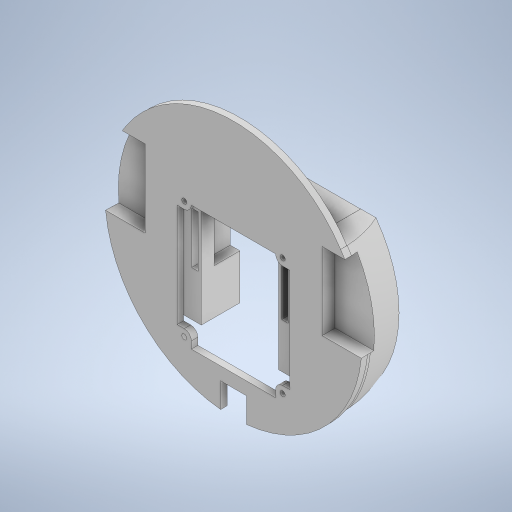
# Autodesk Inventor part: Wabbit
Saved by Autodesk Inventor 2024.2 (Build 282272000, 272)
## iProperties
Created: 2025-11-06
Part Number: Wabbit
Material: Generic
Document SubType Name: Modeling
Designer: David Toler II
Density: 1 g/cm^3
Appearance: Default
Author: David Toler II
Autodesk Inventor part; units mm, degrees
ref_plane "YZ Plane" through (0, 0, 0) normal (1, 0, 0) x (0, 1, 0)
ref_plane "XZ Plane" through (0, 0, 0) normal (0, 1, 0) x (-1, 0, 0)
ref_plane "XY Plane" through (0, 0, 0) normal (0, 0, 1) x (1, 0, 0)
sketch "Sketch1" plane through (0, 0, 0) normal (0, 0, 1) x (1, 0, 0)
  line L0 (27.78125, -44.45) -> (-27.78125, -44.45)
  line L1 (-27.78125, -44.45) -> (-27.78125, 44.45)
  line L2 (-27.78125, 44.45) -> (27.78125, 44.45)
  line L3 (27.78125, 44.45) -> (27.78125, -44.45)
  line L4 (27.78125, -44.45) -> (-27.78125, 44.45) construction
  line L5 (-27.78125, -44.45) -> (27.78125, 44.45) construction
  point P0 (0, 0)
  dimension "d0" = 88.9
  dimension "d1" = 55.5625
  constraints: 12 end point, 2 midpoint, 2 parallel, 1 horizontal, 1 perpendicular
  measures "d0" distance of L0.end L1.end
  measures "d1" distance of L0.start L0.end
extrude "Extrusion1" add sketch "Sketch1" along normal blind 25.4
sketch "Sketch2" plane through (0, 0, 0) normal (1, 0, 0) x (0, 1, 0)
  line L0 (44.45, 0) -> (-44.45, 0)
  line L1 (-44.45, 0) -> (-44.45, 25.4)
  line L2 (44.45, 25.4) -> (-44.45, 25.4)
  line L3 (44.45, 0) -> (44.45, 25.4)
  circle A0 centre (0, 0) radius 63.416389
  line L4 (-63.416389, 0) -> (0, 0)
  line L5 (0, 0) -> (0, 63.416389)
  line L6 (-63.416389, 0) -> (-51.195337, 0)
  line L7 (-54.624765, 25.4) -> (54.624765, 25.4)
  line L8 (54.624765, 25.4) -> (54.624765, 0)
  line L9 (54.624765, 0) -> (-54.624765, 0)
  line L10 (-54.624765, 0) -> (-54.624765, 25.4)
  circle A1 centre (0, 0) radius 60.241389
  line L11 (63.33686, -3.175) -> (-63.33686, -3.175)
  line L12 (0, -3.175) -> (0, 0)
  line L13 (54.624765, 0) -> (63.416389, 0)
  line L14 (-54.624765, 0) -> (-63.416389, 0)
  point P0 (-44.45, 0)
  point P1 (0, 25.4)
  point P2 (44.45, 0)
  dimension "d6" = 109.24953
  dimension "d7" = 3.175
  dimension "d12" = 3.175
  constraints: 22 end point, 6 point on circle, 4 midpoint, 3 perpendicular, 3 point on line, 2 collinear, 2 horizontal, 2 parallel, 1 centre point, 1 coincident, 1 vertical, 3 other
  measures "d6" distance between parallel lines of L8 L10
  measures "d12" distance between parallel lines of L11 L0
revolve "Revolution1" add sketch "Sketch2" angle 360 about axis through (0, 0, 0) along (0, 0, 1) contours L9 L13 A1 L11 L12 L0 | L13 A0 L11 A1
sketch "Sketch6" plane through (0, 0, 0) normal (0, 0, 1) x (1, 0, 0)
  circle A0 centre (0, 0) radius 63.416389
  line L0 (27.78125, -44.45) -> (27.78125, 44.45)
  line L1 (-27.78125, -44.45) -> (27.78125, -44.45)
  line L2 (-27.78125, 44.45) -> (-27.78125, -44.45)
  line L3 (27.78125, 44.45) -> (-27.78125, 44.45)
  line L4 (24.28125, -40.95) -> (24.28125, 40.95)
  line L5 (24.28125, 40.95) -> (-24.28125, 40.95)
  line L6 (-24.28125, 40.95) -> (-24.28125, -40.95)
  line L7 (-24.28125, -40.95) -> (24.28125, -40.95)
  circle A1 centre (-24.28125, -40.95) radius 1.25
  circle A2 centre (24.28125, -40.95) radius 1.25
  line L8 (-24.28125, 17.05) -> (24.28125, 17.05)
  circle A3 centre (-24.28125, 17.05) radius 1.25
  circle A4 centre (24.28125, 17.05) radius 1.25
  circle A5 centre (-24.28125, 17.05) radius 3.5
  circle A6 centre (-24.28125, -40.95) radius 3.5
  circle A7 centre (24.28125, -40.95) radius 3.5
  circle A8 centre (24.28125, 17.05) radius 3.5
  line L9 (-24.28125, 20.55) -> (-27.78125, 20.55)
  line L10 (-24.28125, 13.55) -> (-27.78125, 13.55)
  line L11 (-20.78125, -40.95) -> (-20.78125, -44.45)
  line L12 (-24.28125, -37.45) -> (-27.78125, -37.45)
  line L13 (20.78125, -40.95) -> (20.78125, -44.45)
  line L14 (24.28125, -37.45) -> (27.78125, -37.45)
  line L15 (24.28125, 20.55) -> (27.78125, 20.55)
  line L16 (24.28125, 13.55) -> (27.78125, 13.55)
  point P0 (20.78125, 17.05)
  point P1 (-20.78125, 17.05)
  dimension "d13" = 3.5
  dimension "d14" = 2.5
  dimension "d15" = 2.5
  dimension "d16" = 58
  dimension "d17" = 2.5
  dimension "d18" = 2.5
  constraints: 26 end point, 21 point on line, 8 centre point, 8 point on circle, 8 tangent, 6 perpendicular, 4 coincident, 3 other
  measures "d13" distance between parallel lines of L1 L7
  measures "d14" diameter of A1
  measures "d15" diameter of A2
  measures "d16" distance between parallel lines of L7 L8
  measures "d17" diameter of A3
  measures "d18" diameter of A4
extrude "Extrusion3" cut sketch "Sketch6" along normal through all both and the other way through all contours L14 L4 L16 L0 | A7 L7 A6 L6 A5 L8 A8 L4 | L1 L11 L7 L13 | A2 L7 L4 | L4 L7 A2 | A4 L8 L4 | L4 A4 | A1 L6 L7 | L7 L6 A1 | L12 L2 L10 L6 | L8 A4 L4 | A3 L6 L8 | L8 L6 A3 | A3 L6
sketch "Sketch7" plane through (0, 0, 0) normal (0, 1, 0) x (-1, 0, 0)
  line L0 (-20.78125, -3.175) -> (20.78125, -3.175)
  line L1 (-20.78125, -3.175) -> (-20.78125, 25.4)
  line L2 (20.78125, 25.4) -> (-20.78125, 25.4)
  line L3 (20.78125, -3.175) -> (20.78125, 25.4)
  line L4 (20.78125, 0) -> (20.78125, 25.4)
  line L5 (27.78125, 25.4) -> (20.78125, 25.4)
  line L6 (27.78125, 0) -> (27.78125, 25.4)
  line L7 (27.78125, 0) -> (20.78125, 0)
  line L8 (-20.78125, 25.4) -> (-20.78125, 0)
  line L9 (-20.78125, 0) -> (-27.78125, 0)
  line L10 (-27.78125, 0) -> (-27.78125, 25.4)
  line L11 (-20.78125, 25.4) -> (-27.78125, 25.4)
  line L12 (20.78125, 0) -> (-20.78125, 0)
  point P0 (0, 0)
  constraints: 2 end point, 1 perpendicular
extrude "Extrusion4" cut sketch "Sketch7" along normal through all both and the other way through all contours L9 L10 L11 L1 | L1 L2 L3 L12 | L3 L5 L6 L7
sketch "Sketch8" plane through (0, 0, 0) normal (0, 0, 1) x (1, 0, 0)
  circle A0 centre (-24.28125, -40.95) radius 1.25
  circle A1 centre (-24.28125, 17.05) radius 1.25
  circle A2 centre (24.28125, 17.05) radius 1.25
  circle A3 centre (24.28125, -40.95) radius 1.25
  circle A4 centre (0, 0) radius 63.416389
  line L0 (-24.28125, 13.55) -> (-27.78125, 13.55)
  arc A5 (-24.28125, 13.55) -> (-20.78125, 17.05) centre (-24.28125, 17.05) ccw
  line L1 (20.78125, 17.05) -> (-20.78125, 17.05)
  arc A6 (20.78125, 17.05) -> (24.28125, 13.55) centre (24.28125, 17.05) ccw
  line L2 (27.78125, 13.55) -> (24.28125, 13.55)
  line L3 (27.78125, -37.45) -> (27.78125, 13.55)
  line L4 (24.28125, -37.45) -> (27.78125, -37.45)
  arc A7 (24.28125, -37.45) -> (20.78125, -40.95) centre (24.28125, -40.95) ccw
  line L5 (20.78125, -44.45) -> (20.78125, -40.95)
  line L6 (-20.78125, -44.45) -> (20.78125, -44.45)
  line L7 (-20.78125, -40.95) -> (-20.78125, -44.45)
  arc A8 (-20.78125, -40.95) -> (-24.28125, -37.45) centre (-24.28125, -40.95) ccw
  line L8 (-27.78125, -37.45) -> (-24.28125, -37.45)
  line L9 (-27.78125, 13.55) -> (-27.78125, -37.45)
  circle A9 centre (0, 0) radius 63.33686
  line L10 (-43.632893, 31.829375) -> (-54.758093, 31.829375)
  line L11 (-54.758093, 31.829375) -> (-54.758093, -31.829375)
  line L12 (-54.758093, -31.829375) -> (-43.632893, -31.829375)
  line L13 (-43.632893, -31.829375) -> (-43.632893, 31.829375)
  line L14 (-43.632893, 31.829375) -> (-54.758093, -31.829375) construction
  line L15 (-54.758093, 31.829375) -> (-43.632893, -31.829375) construction
  line L16 (43.737562, 31.670625) -> (54.850062, 31.670625)
  line L17 (54.850062, 31.670625) -> (54.850062, -31.829375)
  line L18 (54.850062, -31.829375) -> (43.737562, -31.829375)
  line L19 (43.737562, -31.829375) -> (43.737562, 31.670625)
  line L20 (43.737562, 31.670625) -> (54.850062, -31.829375) construction
  line L21 (54.850062, 31.670625) -> (43.737562, -31.829375) construction
  line L22 (43.737562, -6.429375) -> (54.850062, -6.429375)
  line L23 (-43.632893, -6.270625) -> (-54.758093, -6.270625)
  line L24 (-54.758093, -6.270625) -> (-63.025686, -6.270625)
  line L25 (54.850062, -6.429375) -> (63.009689, -6.429375)
  point P0 (-49.195493, 0)
  point P1 (49.293812, -0.079375)
  point P2 (54.758093, -31.829375)
  dimension "d23" = 63.5
  dimension "d24" = 11.1125
  dimension "d25" = 11.1252
  dimension "d35" = 38.1
  dimension "d36" = 38.1
  constraints: 32 end point, 5 point on circle, 5 point on line, 4 horizontal, 4 midpoint, 4 parallel, 4 perpendicular, 2 other
  measures "d23" distance of L16.end L17.end
  measures "d24" distance of L16.start L16.end
  measures "d25" distance of L10.start L10.end
  measures "d35" distance between parallel lines of L22 L16
  measures "d36" distance between parallel lines of L23 L10
extrude "Extrusion5" cut sketch "Sketch8" against normal through all contours L25 L17 A9 | L22 L19 L16 L17 | A9 L11 L24 | L11 L10 L13 L23 picked at (56.405575, 15.635107) picked at (-56.188118, 16.156275)
sketch "Sketch9" plane through (43.737562, -31.829375, 0) normal (1, 0, 0) x (0, 0, -1)
  line L0 (3.175, 63.5) -> (3.175, 25.4) projected
  line L1 (0, 63.5) -> (3.175, 63.5) projected
  line L2 (0, 25.4) -> (0, 63.5) projected
  line L3 (0, 25.4) -> (3.175, 25.4) projected
  line L4 (3.175, 25.4) -> (3.175, 63.5) projected
  line L5 (0, 25.4) -> (3.175, 25.4) projected
  line L6 (0, 63.5) -> (0, 25.4) projected
  line L7 (0, 63.5) -> (3.175, 63.5) projected
  point P0 (0, 31.829375)
extrude "Extrusion6" cut sketch "Sketch9" along normal blind 25.4
sketch "Sketch10" plane through (-43.632893, -31.829375, 0) normal (-1, 0, 0) x (0, 0, 1)
  line L0 (-3.175, 25.55875) -> (-3.175, 63.65875)
  line L1 (0, 63.65875) -> (0, 25.55875)
  line L2 (0, 63.65875) -> (-3.175, 63.65875)
  line L3 (0, 25.55875) -> (-3.175, 25.55875)
  point P0 (0, 31.829375)
extrude "Extrusion7" cut sketch "Sketch10" along normal through all
sketch "Sketch12" plane through (-63.105608, -6.270625, 0) normal (0, 0, 1) x (1, 0, 0)
  line L0 (19.472715, 0) -> (0, 0)
  arc A0 (0, 0) -> (126.195239, -0.15875) centre (63.105608, 6.270625) ccw
  line L1 (126.195239, -0.15875) -> (106.84317, -0.15875)
  line L2 (106.84317, -0.15875) -> (106.84317, 37.94125)
  line L3 (106.84317, 37.94125) -> (118.047486, 37.94125)
  arc A1 (118.047486, 37.94125) -> (8.255545, 38.1) centre (63.105608, 6.270625) ccw
  line L4 (8.255545, 38.1) -> (19.472715, 38.1)
  line L5 (19.472715, 38.1) -> (19.472715, 0)
  circle A2 centre (38.824358, -34.679375) radius 1.25
  circle A3 centre (38.824358, 23.320625) radius 1.25
  circle A4 centre (87.386858, 23.320625) radius 1.25
  circle A5 centre (87.386858, -34.679375) radius 1.25
  line L6 (38.824358, 19.820625) -> (35.324358, 19.820625)
  arc A6 (38.824358, 19.820625) -> (42.324358, 23.320625) centre (38.824358, 23.320625) ccw
  line L7 (83.886858, 23.320625) -> (42.324358, 23.320625)
  arc A7 (83.886858, 23.320625) -> (87.386858, 19.820625) centre (87.386858, 23.320625) ccw
  line L8 (90.886858, 19.820625) -> (87.386858, 19.820625)
  line L9 (90.886858, -31.179375) -> (90.886858, 19.820625)
  line L10 (87.386858, -31.179375) -> (90.886858, -31.179375)
  arc A8 (87.386858, -31.179375) -> (83.886858, -34.679375) centre (87.386858, -34.679375) ccw
  line L11 (83.886858, -38.179375) -> (83.886858, -34.679375)
  line L12 (42.324358, -38.179375) -> (83.886858, -38.179375)
  line L13 (42.324358, -34.679375) -> (42.324358, -38.179375)
  arc A9 (42.324358, -34.679375) -> (38.824358, -31.179375) centre (38.824358, -34.679375) ccw
  line L14 (35.324358, -31.179375) -> (38.824358, -31.179375)
  line L15 (35.324358, 19.820625) -> (35.324358, -31.179375)
  arc A10 (0.079922, 0) -> (126.115297, -0.15875) centre (63.105608, 6.270625) ccw
  line L16 (125.734179, -3.175) -> (103.66817, -3.175)
  line L17 (103.66817, -3.175) -> (103.66817, 41.275)
  line L18 (103.66817, 41.275) -> (115.985965, 41.275)
  line L19 (0.477036, -3.175) -> (22.647715, -3.175)
  line L20 (22.647715, -3.175) -> (22.647715, 41.275)
  line L21 (22.647715, 41.275) -> (10.22525, 41.275)
  dimension "d39" = 3.175
  dimension "d40" = 3.175
  dimension "d41" = 3.175
  dimension "d42" = 3.175
  constraints: 12 end point, 4 point on circle, 4 point on line, 3 perpendicular, 1 horizontal
  measures "d39" distance between parallel lines of L0 L19
  measures "d40" distance between parallel lines of L5 L20
  measures "d41" distance between parallel lines of L4 L21
  measures "d42" distance between parallel lines of L17 L2
extrude "Extrusion9" add sketch "Sketch12" against normal blind 6.35 contours L5 L4 A1 L21 L20 L19 A10 L0 | L16 L17 L18 A1 L3 L2 L1 A10
sketch "Sketch16" plane through (-63.105608, -6.270625, -6.35) normal (0, 0, -1) x (-1, 0, 0)
  line L0 (-0.079922, 0) -> (-19.472715, 0)
  line L1 (-19.472715, 0) -> (-19.472715, 38.1)
  line L2 (-19.472715, 38.1) -> (-8.255545, 38.1)
  arc A0 (-8.255545, 38.1) -> (-10.22525, 41.275) centre (-63.105608, 6.270625) ccw
  line L3 (-10.22525, 41.275) -> (-22.647715, 41.275)
  line L4 (-22.647715, 41.275) -> (-22.647715, -3.175)
  line L5 (-22.647715, -3.175) -> (-0.477036, -3.175)
  arc A1 (-0.477036, -3.175) -> (-0.079922, 0) centre (-63.105608, 6.270625) ccw
  line L6 (-22.647715, 41.275) -> (-10.320652, 41.275)
  arc A2 (-10.320652, 41.275) -> (-115.890563, 41.275) centre (-63.105608, 6.270625) ccw
  line L7 (-115.890563, 41.275) -> (-103.66817, 41.275)
  line L8 (-103.66817, 41.275) -> (-103.66817, -3.175)
  line L9 (-103.66817, -3.175) -> (-125.734179, -3.175)
  arc A3 (-125.734179, -3.175) -> (-0.477036, -3.175) centre (-63.105608, 6.270625) ccw
  line L10 (-0.477036, -3.175) -> (-22.647715, -3.175)
  line L11 (-22.647715, -3.175) -> (-22.647715, 41.275)
  circle A4 centre (-87.386858, -34.679375) radius 1.25
  circle A5 centre (-87.386858, 23.320625) radius 1.25
  circle A6 centre (-38.824358, -34.679375) radius 1.25
  circle A7 centre (-38.824358, 23.320625) radius 1.25
  line L12 (-83.886858, -38.179375) -> (-83.886858, -34.679375)
  arc A8 (-83.886858, -34.679375) -> (-87.386858, -31.179375) centre (-87.386858, -34.679375) ccw
  line L13 (-87.386858, -31.179375) -> (-90.886858, -31.179375)
  line L14 (-90.886858, -31.179375) -> (-90.886858, 19.820625)
  line L15 (-90.886858, 19.820625) -> (-87.386858, 19.820625)
  arc A9 (-87.386858, 19.820625) -> (-83.886858, 23.320625) centre (-87.386858, 23.320625) ccw
  line L16 (-83.886858, 23.320625) -> (-42.324358, 23.320625)
  arc A10 (-42.324358, 23.320625) -> (-38.824358, 19.820625) centre (-38.824358, 23.320625) ccw
  line L17 (-38.824358, 19.820625) -> (-35.324358, 19.820625)
  line L18 (-35.324358, 19.820625) -> (-35.324358, -31.179375)
  line L19 (-35.324358, -31.179375) -> (-38.824358, -31.179375)
  arc A11 (-38.824358, -31.179375) -> (-42.324358, -34.679375) centre (-38.824358, -34.679375) ccw
  line L20 (-42.324358, -34.679375) -> (-42.324358, -38.179375)
  line L21 (-42.324358, -38.179375) -> (-83.886858, -38.179375)
  arc A12 (-115.985965, 41.275) -> (-118.047486, 37.94125) centre (-63.105608, 6.270625) ccw
  line L22 (-118.047486, 37.94125) -> (-106.84317, 37.94125)
  line L23 (-106.84317, 37.94125) -> (-106.84317, -0.15875)
  line L24 (-106.84317, -0.15875) -> (-126.115297, -0.15875)
  arc A13 (-126.115297, -0.15875) -> (-125.734179, -3.175) centre (-63.105608, 6.270625) ccw
  line L25 (-125.734179, -3.175) -> (-103.66817, -3.175)
  line L26 (-103.66817, -3.175) -> (-103.66817, 41.275)
  line L27 (-103.66817, 41.275) -> (-115.985965, 41.275)
  circle A14 centre (-63.105608, 6.270625) radius 63.33686
  point P0 (-117.95567, 37.94125)
  point P1 (-126.115297, -0.15875)
  point P2 (-115.890563, 41.275)
  point P3 (-10.320652, 41.275)
  constraints: 1 coincident, 3 other
extrude "Extrusion12" add sketch "Sketch16" along normal blind 3.175 contours A1 L5 L4 L3 A14 L2 L1 L0 | L0 L1 L2 A14 | A13 L24 L23 L22 A14 L7 L8 L9 | A14 L22 L23 L24 | L22 A12 L27 A14
sketch "Sketch17" plane through (0, 0, -3.175) normal (0, 0, -1) x (-1, 0, 0)
  line L0 (40.457893, 35.004375) -> (52.784956, 35.004375)
  arc A0 (52.784956, 35.004375) -> (-52.784956, 35.004375) centre (0, 0) ccw
  line L1 (-52.784956, 35.004375) -> (-40.562562, 35.004375)
  line L2 (-40.562562, 35.004375) -> (-40.562562, -9.445625)
  line L3 (-40.562562, -9.445625) -> (-62.628572, -9.445625)
  arc A1 (-62.628572, -9.445625) -> (62.628572, -9.445625) centre (0, 0) ccw
  line L4 (62.628572, -9.445625) -> (40.457893, -9.445625)
  line L5 (40.457893, -9.445625) -> (40.457893, 35.004375)
  circle A2 centre (-24.28125, -40.95) radius 1.25
  circle A3 centre (-24.28125, 17.05) radius 1.25
  circle A4 centre (24.28125, -40.95) radius 1.25
  circle A5 centre (24.28125, 17.05) radius 1.25
  line L6 (-20.78125, -44.45) -> (-20.78125, -40.95)
  arc A6 (-20.78125, -40.95) -> (-24.28125, -37.45) centre (-24.28125, -40.95) ccw
  line L7 (-24.28125, -37.45) -> (-27.78125, -37.45)
  line L8 (-27.78125, -37.45) -> (-27.78125, 13.55)
  line L9 (-27.78125, 13.55) -> (-24.28125, 13.55)
  arc A7 (-24.28125, 13.55) -> (-20.78125, 17.05) centre (-24.28125, 17.05) ccw
  line L10 (-20.78125, 17.05) -> (20.78125, 17.05)
  arc A8 (20.78125, 17.05) -> (24.28125, 13.55) centre (24.28125, 17.05) ccw
  line L11 (24.28125, 13.55) -> (27.78125, 13.55)
  line L12 (27.78125, 13.55) -> (27.78125, -37.45)
  line L13 (27.78125, -37.45) -> (24.28125, -37.45)
  arc A9 (24.28125, -37.45) -> (20.78125, -40.95) centre (24.28125, -40.95) ccw
  line L14 (20.78125, -40.95) -> (20.78125, -44.45)
  line L15 (20.78125, -44.45) -> (-20.78125, -44.45)
  circle A10 centre (0, 0) radius 63.33686
  line L16 (-19.05, -60.4041) -> (19.05, -60.4041)
  line L17 (19.05, -60.4041) -> (19.05, 60.4041)
  line L18 (19.05, 60.4041) -> (-19.05, 60.4041)
  line L19 (-19.05, 60.4041) -> (-19.05, -60.4041)
  line L20 (-19.05, -60.4041) -> (19.05, 60.4041) construction
  line L21 (19.05, -60.4041) -> (-19.05, 60.4041) construction
  arc A11 (-62.628572, -9.445625) -> (62.628572, -9.445625) centre (0, 0) ccw
  line L22 (-52.837507, 34.925) -> (52.837507, 34.925)
  line L23 (52.837507, 34.925) -> (52.837507, -34.925)
  line L24 (52.837507, -34.925) -> (-52.837507, -34.925)
  line L25 (-52.837507, -34.925) -> (-52.837507, 34.925)
  line L26 (-52.837507, 34.925) -> (52.837507, -34.925) construction
  line L27 (52.837507, 34.925) -> (-52.837507, -34.925) construction
  point P0 (0, 0)
  point P1 (52.837507, -34.925)
  point P2 (40.457893, 34.925)
  point P3 (19.05, 34.925)
  point P4 (19.05, -34.925)
  point P5 (-19.05, 34.925)
  point P6 (-40.562562, 34.925)
  point P7 (-19.05, -34.925)
  dimension "d53" = 69.85
  dimension "d54" = 38.1
  constraints: 24 end point, 4 midpoint, 4 parallel, 3 point on circle, 2 horizontal, 2 perpendicular, 1 centre point, 1 coincident
  measures "d53" distance between parallel lines of L24 L22
  measures "d54" distance between parallel lines of L19 L17
extrude "Extrusion13" add sketch "Sketch17" along normal blind 6.35 contours L5 L4 L23 L24 L12 L11 A8 L10 L17 L22 | L4 A1 L23 | L10 A8 L11 L12 L24 L17 | L19 L10 A7 L9 L8 L24 L25 L3 L2 L22 | L19 L24 L8 L9 A7 L10 | L3 L25 A1
sketch "Sketch18" plane through (-63.105608, -6.270625, -9.525) normal (0, 0, -1) x (-1, 0, 0)
  circle A0 centre (-38.824358, 23.320625) radius 1.25
  line L0 (-10.320652, 41.275) -> (-22.647715, 41.275)
  line L1 (-22.647715, 41.275) -> (-22.647715, 41.195625)
  line L2 (-22.647715, 41.195625) -> (-44.055608, 41.195625)
  line L3 (-44.055608, 41.195625) -> (-44.055608, -28.654375)
  line L4 (-44.055608, -28.654375) -> (-10.2681, -28.654375)
  arc A1 (-10.2681, -28.654375) -> (-10.320652, 41.275) centre (-63.105608, 6.270625) ccw
  circle A2 centre (-87.386858, 23.320625) radius 1.25
  arc A3 (-117.95567, 37.94125) -> (-115.943115, -28.654375) centre (-63.105608, 6.270625) ccw
  line L5 (-115.943115, -28.654375) -> (-82.155608, -28.654375)
  line L6 (-82.155608, -28.654375) -> (-82.155608, 41.195625)
  line L7 (-82.155608, 41.195625) -> (-103.66817, 41.195625)
  line L8 (-103.66817, 41.195625) -> (-103.66817, 41.275)
  line L9 (-103.66817, 41.275) -> (-115.985965, 41.275)
  arc A4 (-115.985965, 41.275) -> (-118.047486, 37.94125) centre (-63.105608, 6.270625) ccw
  line L10 (-118.047486, 37.94125) -> (-117.95567, 37.94125)
  line L11 (-63.105608, 6.270625) -> (0.231234, 6.318222)
  arc A5 (-0.079922, 0) -> (-8.347515, 38.1) centre (-63.105608, 6.270625) ccw
  line L12 (-63.105608, 6.270625) -> (-126.44245, 6.223028)
  line L13 (-39.293108, 18.987327) -> (-42.468108, 18.987327)
  line L14 (-42.468108, 18.987327) -> (-42.468108, -6.412673)
  line L15 (-42.468108, -6.412673) -> (-39.293108, -6.412673)
  line L16 (-39.293108, -6.412673) -> (-39.293108, 18.987327)
  line L17 (-39.293108, 18.987327) -> (-42.468108, -6.412673) construction
  line L18 (-42.468108, 18.987327) -> (-39.293108, -6.412673) construction
  line L19 (-63.105608, 6.270625) -> (-63.105608, 69.607485)
  arc A6 (-10.320652, 41.275) -> (-115.890563, 41.275) centre (-63.105608, 6.270625) ccw
  line L20 (-86.918108, 18.987327) -> (-83.743108, 18.987327)
  line L21 (-83.743108, 18.987327) -> (-83.743108, -6.412673)
  line L22 (-83.743108, -6.412673) -> (-86.918108, -6.412673)
  line L23 (-86.918108, -6.412673) -> (-86.918108, 18.987327)
  point P0 (-40.880608, 6.287327)
  dimension "d57" = 3.175
  dimension "d58" = 25.4
  dimension "d59" = 3.175
  constraints: 26 end point, 4 point on circle, 4 symmetric about line, 2 midpoint, 2 parallel, 2 point on line, 1 horizontal, 1 perpendicular, 1 vertical
  measures "d57" distance between parallel lines of L14 L16
  measures "d58" distance of L13.end L14.end
  measures "d59" distance from line of L3 point (-40.881, 6.287)
extrude "Extrusion14" cut sketch "Sketch18" against normal blind 6.35 contours L16 L15 L14 L11 | L11 L14 L13 L16 | L21 L22 L23 L12 | L12 L23 L20 L21
sketch "Sketch20" plane through (0, 0, -3.175) normal (0, 0, -1) x (-1, 0, 0)
  line L0 (19.05, 34.925) -> (40.457893, 34.925)
  line L1 (40.457893, 34.925) -> (40.457893, 35.004375)
  line L2 (40.457893, 35.004375) -> (52.784956, 35.004375)
  arc A0 (52.784956, 35.004375) -> (-52.784956, 35.004375) centre (0, 0) ccw
  line L3 (-52.784956, 35.004375) -> (-40.562562, 35.004375)
  line L4 (-40.562562, 35.004375) -> (-40.562562, 34.925)
  line L5 (-40.562562, 34.925) -> (-19.05, 34.925)
  line L6 (-19.05, 34.925) -> (-19.05, 17.05)
  line L7 (-19.05, 17.05) -> (19.05, 17.05)
  line L8 (19.05, 17.05) -> (19.05, 34.925)
  line L9 (19.05, 34.925) -> (-19.05, 34.925)
  line L10 (-19.05, 34.925) -> (-19.05, 28.575)
  line L11 (-19.05, 28.575) -> (19.05, 28.575)
  line L12 (19.05, 28.575) -> (19.05, 34.925)
  point P0 (19.05, 28.575)
  dimension "d65" = 6.35
  constraints: 8 end point, 2 parallel, 1 horizontal, 1 perpendicular, 1 point on line
  measures "d65" distance between parallel lines of L9 L11
extrude "Extrusion15" add sketch "Sketch20" along normal blind 6.35 contours L8 L11 L6 L9
sketch "Sketch19" plane through (0, 0, 0) normal (0, 1, 0) x (-1, 0, 0)
  circle A0 centre (0, 0) radius 63.5
  circle A1 centre (0, 0) radius 76.2
  line L0 (76.2, 0) -> (63.5, 0)
  line L1 (-63.5, 0) -> (-76.2, 0)
  line L2 (0, 0) -> (0, -76.2)
  line L3 (52.837507, -3.175) -> (-52.837507, -3.175)
  line L4 (0, 0) -> (-63.5, 0)
  line L5 (0, 0) -> (63.5, 0)
  point P0 (0, -63.5)
  dimension "d62" = 127
  dimension "d63" = 152.4
  constraints: 10 end point, 5 point on circle, 2 centre point, 2 coincident, 2 perpendicular, 1 collinear, 1 horizontal, 1 point on line
  measures "d62" diameter of A0
  measures "d63" diameter of A1
revolve "Revolution2" cut sketch "Sketch19" angle 360 about axis through (0, 0, 0) along (0, 0, -1) contours A0 L2 A1 L1
sketch "Sketch21" plane through (-63.105608, -6.270625, -9.525) normal (0, 0, -1) x (-1, 0, 0)
  arc A0 (-115.222957, 41.275) -> (-115.276181, -28.654375) centre (-63.105608, 6.270625) ccw
  line L0 (-115.276181, -28.654375) -> (-82.155608, -28.654375)
  line L1 (-82.155608, -28.654375) -> (-82.155608, 34.845625)
  line L2 (-82.155608, 34.845625) -> (-44.055608, 34.845625)
  line L3 (-44.055608, 34.845625) -> (-44.055608, -28.654375)
  line L4 (-44.055608, -28.654375) -> (-10.935034, -28.654375)
  arc A1 (-10.935034, -28.654375) -> (-10.988258, 41.275) centre (-63.105608, 6.270625) ccw
  line L5 (-10.988258, 41.275) -> (-22.647715, 41.275)
  line L6 (-22.647715, 41.275) -> (-22.647715, 41.195625)
  line L7 (-22.647715, 41.195625) -> (-103.66817, 41.195625)
  line L8 (-103.66817, 41.195625) -> (-103.66817, 41.275)
  line L9 (-103.66817, 41.275) -> (-115.222957, 41.275)
  circle A2 centre (-38.824358, 23.320625) radius 1.25
  line L10 (-39.293108, -6.412673) -> (-42.468108, -6.412673)
  line L11 (-42.468108, -6.412673) -> (-42.468108, 18.987327)
  line L12 (-42.468108, 18.987327) -> (-39.293108, 18.987327)
  line L13 (-39.293108, 18.987327) -> (-39.293108, -6.412673)
  line L14 (-86.918108, 18.987327) -> (-83.743108, 18.987327)
  line L15 (-83.743108, 18.987327) -> (-83.743108, -6.412673)
  line L16 (-83.743108, -6.412673) -> (-86.918108, -6.412673)
  line L17 (-86.918108, -6.412673) -> (-86.918108, 18.987327)
  circle A3 centre (-87.386858, 23.320625) radius 1.25
  line L18 (-42.468108, 18.987327) -> (-44.055608, 18.987327)
  line L19 (-42.468108, -6.412673) -> (-44.055608, -6.412673)
  line L20 (-83.743108, 18.987327) -> (-82.155608, 18.987327)
  line L21 (-83.743108, -6.412673) -> (-82.155608, -6.412673)
  constraints: 8 end point, 6 point on line, 2 perpendicular
extrude "Extrusion16" add sketch "Sketch21" along normal blind 12.7 contours L9 L8 L7 L6 L5 A1 L4 L3 L19 L10 L13 L12 L18 L2 L1 L20 L14 L17 L16 L21 L0 A0
sketch "Sketch22" plane through (0, 0, 0) normal (0, 1, 0) x (-1, 0, 0)
  circle A0 centre (0, 0) radius 63.5
  circle A1 centre (0, 0) radius 76.2
  line L0 (76.2, 0) -> (63.5, 0)
  line L1 (-63.5, 0) -> (-76.2, 0)
  line L2 (0, 0) -> (0, -76.2)
  line L3 (0, 0) -> (-63.5, 0)
  line L4 (0, 0) -> (63.5, 0)
  line L5 (52.880357, 0) -> (-52.880357, 0)
  line L6 (0, 0) -> (76.2, 0)
  point P0 (0, 0)
  point P1 (57.799681, -33.868519)
  point P2 (0, -63.5)
  dimension "d70" = 127
  dimension "d71" = 152.4
  constraints: 12 end point, 6 point on circle, 3 coincident, 3 point on line, 2 centre point, 1 collinear, 1 horizontal, 1 midpoint, 1 perpendicular
  measures "d70" diameter of A0
  measures "d71" diameter of A1
revolve "Revolution3" cut sketch "Sketch22" angle 360 about axis through (0, 0, 0) along (0, 0, -1) contours L0 A1 L2 A0
sketch "Sketch23" plane through (20.78125, -44.45, -3.175) normal (0, 0, -1) x (-1, 0, 0)
  circle A0 centre (45.0625, 3.5) radius 1.25
  circle A1 centre (-3.5, 3.5) radius 1.25
  line L0 (73.618757, 9.525) -> (48.5625, 9.525)
  line L1 (48.5625, 9.525) -> (48.5625, 7)
  line L2 (48.5625, 7) -> (45.0625, 7)
  arc A2 (45.0625, 7) -> (41.5625, 3.5) centre (45.0625, 3.5) ccw
  line L3 (41.5625, 3.5) -> (41.5625, 0)
  line L4 (41.5625, 0) -> (0, 0)
  line L5 (0, 0) -> (0, 3.5)
  arc A3 (0, 3.5) -> (-3.5, 7) centre (-3.5, 3.5) ccw
  line L6 (-3.5, 7) -> (-7, 7)
  line L7 (-7, 7) -> (-7, 9.525)
  line L8 (-7, 9.525) -> (-32.056257, 9.525)
  arc A4 (-32.056257, 9.525) -> (73.618757, 9.525) centre (20.78125, 44.45) ccw
  line L9 (41.5625, 0) -> (0, 0)
  line L10 (20.78125, 0) -> (20.78125, -18.88686)
  line L11 (27.13125, -31.42372) -> (14.43125, -31.42372)
  line L12 (14.43125, -31.42372) -> (14.43125, -6.35)
  line L13 (14.43125, -6.35) -> (27.13125, -6.35)
  line L14 (27.13125, -6.35) -> (27.13125, -31.42372)
  line L15 (27.13125, -31.42372) -> (14.43125, -6.35) construction
  line L16 (14.43125, -31.42372) -> (27.13125, -6.35) construction
  arc A5 (-32.056257, 9.525) -> (73.618757, 9.525) centre (20.78125, 44.45) ccw
  point P0 (20.78125, -18.88686)
  dimension "d73" = 6.35
  dimension "d74" = 12.7
  constraints: 14 end point, 3 midpoint, 2 parallel, 2 point on circle, 1 horizontal, 1 perpendicular, 1 point on line
  measures "d73" distance between parallel lines of L4 L13
  measures "d74" distance between parallel lines of L12 L14
extrude "Extrusion17" cut sketch "Sketch23" against normal blind 12.7 contours L14 L11 L12 A4 | A4 L10 L13 L14 | A4 L12 L13 L10
body "Solid1"
